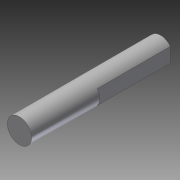
# Autodesk Inventor part: Axis
Saved by Autodesk Inventor 2014 SP1 (Build 180222100, 222)
## iProperties
Created: 2017-07-08
Part Number: Axis
Material: Типовые
Document SubType Name: Modeling
Designer: Stepan
Density: 1 g/cm^3
Appearance: Сталь
Author: Stepan
Autodesk Inventor part; units mm, degrees
ref_plane "YZ Plane" through (0, 0, 0) normal (1, 0, 0) x (0, 1, 0)
ref_plane "XZ Plane" through (0, 0, 0) normal (0, 1, 0) x (-1, 0, 0)
ref_plane "XY Plane" through (0, 0, 0) normal (0, 0, 1) x (1, 0, 0)
sketch "Эскиз1" plane through (0, 0, 0) normal (0, 1, 0) x (-1, 0, 0)
  circle A0 centre (0, 0) radius 2.5
  dimension "d0" = 5
  constraints: 1 centre point, 1 coincident
  measures "d0" diameter of A0
extrude "Выдавливание1" add sketch "Эскиз1" along normal blind 29
sketch "Эскиз2" plane through (0, 29, 0) normal (0, 1, 0) x (1, 0, 0)
  circle A0 centre (0, 0) radius 2.5 projected
  line L0 (-2.5, 0) -> (2, 0)
  line L1 (2, 0) -> (2, 1.5)
  line L2 (2, 0) -> (2, -1.5)
  dimension "d3" = 4.5
  constraints: 6 end point, 3 point on circle, 1 collinear, 1 horizontal, 1 perpendicular
  measures "d3" distance of L0.start L0.end
extrude "Выдавливание2" cut sketch "Эскиз2" against normal blind 15 contours A0 L2 L1
